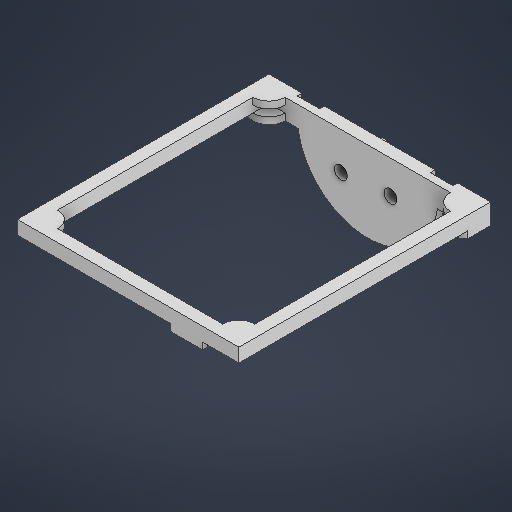
# Autodesk Inventor part: Frame
Saved by Autodesk Inventor 2026.1 (Build 301233020, 233B)
## iProperties
Created: 2026-09-21
Part Number: Frame
Material: Generic
Document SubType Name: Modeling
Designer: InventorKid
Density: 1 g/cm^3
Appearance: Default
Author: InventorKid
Autodesk Inventor part; units mm, degrees
ref_plane "YZ Plane" through (0, 0, 0) normal (1, 0, 0) x (0, 1, 0)
ref_plane "XZ Plane" through (0, 0, 0) normal (0, 1, 0) x (-1, 0, 0)
ref_plane "XY Plane" through (0, 0, 0) normal (0, 0, 1) x (1, 0, 0)
sketch "Sketch1" plane through (0, 0, 0) normal (0, 1, 0) x (-1, 0, 0)
  line L0 (0, 0) -> (48.5, 0)
  line L1 (48.5, 0) -> (48.5, 56)
  line L2 (48.5, 56) -> (0, 56)
  line L3 (0, 56) -> (0, 0)
  line L4 (48.8, 56.3) -> (48.8, -0.3)
  line L5 (48.8, -0.3) -> (-0.3, -0.3)
  line L6 (-0.3, -0.3) -> (-0.3, 56.3)
  line L7 (-0.3, 56.3) -> (48.8, 56.3)
  line L8 (51.8, 59.3) -> (51.8, -3.3)
  line L9 (51.8, -3.3) -> (-3.3, -3.3)
  line L10 (-3.3, -3.3) -> (-3.3, 59.3)
  line L11 (-3.3, 59.3) -> (51.8, 59.3)
  dimension "d0" = 56
  dimension "d1" = 48.5
  dimension "d2" = 0.3
  dimension "d3" = 3
  constraints: 24 end point, 6 parallel, 3 perpendicular, 1 horizontal, 6 other
  measures "d0" distance of L0.end L1.end
  measures "d1" distance of L1.end L2.end
  measures "d2" distance between parallel lines of L1 L4
  measures "d3" distance between parallel lines of L7 L11
extrude "Extrusion1" add sketch "Sketch1" along normal blind 1.7 contours L8 L9 L10 L11
sketch "Sketch2" plane through (0, 1.7, 0) normal (0, 1, 0) x (1, 0, 0)
  line L0 (-48.8, 0.3) -> (0.3, 0.3) projected
  line L1 (-51.8, 3.3) -> (-51.8, -59.3) projected
  line L2 (-51.8, -2.3458) -> (-51.8, 3.3)
  line L3 (-51.8, 3.3) -> (-46.1542, 3.3)
  line L4 (-2.3458, 3.3) -> (3.3, 3.3)
  arc A0 (-48.8, -3.7) -> (-44.8, 0.3) centre (-48.8, 0.3) ccw
  line L5 (3.3, -59.3) -> (3.3, 3.3) projected
  line L6 (3.3, -2.3458) -> (3.3, 3.3)
  arc A1 (-3.7, 0.3) -> (0.3, -3.7) centre (0.3, 0.3) ccw
  line L7 (0.3, -56.3) -> (-48.8, -56.3) projected
  arc A2 (-44.8, -56.3) -> (-48.8, -52.3) centre (-48.8, -56.3) ccw
  arc A3 (0.3, -52.3) -> (-3.7, -56.3) centre (0.3, -56.3) ccw
  line L8 (-51.8, -59.3) -> (3.3, -59.3) projected
  line L9 (-2.3458, -59.3) -> (3.3, -59.3)
  line L10 (3.3, -59.3) -> (3.3, -53.6542)
  line L11 (-46.1542, -59.3) -> (-51.8, -59.3)
  line L12 (-51.8, -59.3) -> (-51.8, -53.6542)
  line L13 (-48.8, -56.3) -> (-48.8, 0.3) projected
  line L14 (-44.8, 0.3) -> (-3.7, 0.3)
  line L15 (3.3, 0.3) -> (3.3, 3.3)
  line L16 (3.3, 3.3) -> (-48.8, 3.3)
  line L17 (3.3, -59.3) -> (-51.8, -59.3)
  line L18 (-51.8, -59.3) -> (-51.8, 3.3)
  line L19 (-51.8, 3.3) -> (3.3, 3.3)
  line L20 (3.3, 3.3) -> (3.3, -59.3)
  line L21 (0.3, 0.3) -> (0.3, -56.3) projected
  line L22 (-44.8, 0.3) -> (-3.7, 0.3)
  line L23 (0.3, -3.7) -> (0.3, -52.3)
  line L24 (-3.7, -56.3) -> (-44.8, -56.3)
  line L25 (-48.8, -52.3) -> (-48.8, -3.7)
  point P0 (0, 0)
  point P1 (-48.8, -3.7)
  point P2 (-48.8, -3.7)
  dimension "d8" = 4
  dimension "d9" = 4
  dimension "d14" = 8
  dimension "d15" = 8
  constraints: 38 end point, 8 point on circle, 5 horizontal, 5 parallel, 5 point on line, 4 centre point, 4 perpendicular, 2 coincident, 2 collinear, 1 vertical
  measures "d8" radius of A0
  measures "d9" radius of A1
  measures "d14" diameter of A2
  measures "d15" diameter of A3
extrude "Extrusion2" add sketch "Sketch2" along normal blind 1.7 contours L0 A0 L13 | L0 L21 A1 | A2 L7 L13 | L21 L7 A3 | L3 L16 L4 L5 L8 L1
sketch "Sketch3" plane through (0, 0, 0) normal (0, -1, 0) x (1, 0, 0)
  line L0 (-51.8, 59.3) -> (-51.8, 59.3) projected
  arc A0 (-13.7, 59.3) -> (-5.7, 59.3) centre (-9.7, 59.3) ccw
  line L1 (-13.7, 59.3) -> (-5.7, 59.3)
  arc A1 (-48.8, 52.3) -> (-44.8, 56.3) centre (-48.8, 56.3) ccw projected
  line L2 (0.3, -0.3) -> (0.3, 56.3) projected
  line L3 (3.3, -3.3) -> (-51.8, -3.3) projected
  line L4 (3.3, 59.3) -> (3.3, -3.3) projected
  line L5 (-51.8, -3.3) -> (-51.8, 59.3) projected
  arc A2 (-44.8, -0.3) -> (-48.8, 3.7) centre (-48.8, -0.3) ccw projected
  arc A3 (0.3, 3.7) -> (-3.7, -0.3) centre (0.3, -0.3) ccw projected
  line L6 (-48.8, -0.3) -> (0.3, -0.3) projected
  arc A4 (-46.1542, -3.3) -> (-51.8, 2.3458) centre (-48.8, -0.3) ccw
  arc A5 (3.3, 2.3458) -> (-2.3458, -3.3) centre (0.3, -0.3) ccw
  line L7 (-44.8, -0.3) -> (-3.7, -0.3)
  line L8 (3.3, 2.3458) -> (3.3, -3.3)
  line L9 (-51.8, -3.3) -> (-51.8, 2.3458)
  line L10 (-51.8, 59.3) -> (3.3, 59.3) projected
  dimension "d16" = 4
  dimension "d21" = 10
  constraints: 8 end point, 6 point on circle, 4 collinear, 4 point on line, 3 centre point, 2 coincident, 2 concentric, 2 midpoint, 1 horizontal, 1 other
  measures "d16" radius of A0
  measures "d21" horizontal distance of A0.centre L2.end
extrude "Extrusion3" add sketch "Sketch3" along normal blind 1.7 contours L1 A0 | A4 A2 L3 L5 | L4 L3 A5 L6 L2 | L2 L6 A3 | A4 L6 A5 L3
sketch "Sketch7" plane through (3.3, 3.4, -3.3) normal (0, 0, -1) x (-1, 0, 0)
  line L0 (55.1, -5.1) -> (0, -5.1) construction
  line L1 (0, 0) -> (55.1, 0) construction
  line L2 (55.1, -5.1) -> (0, 0) construction
  line L3 (0, -5.1) -> (55.1, 0) construction
  line L4 (45.05, -5.1) -> (10.05, -5.1)
  line L5 (10.05, -5.1) -> (10.05, 0)
  line L6 (10.05, 0) -> (45.05, 0)
  line L7 (45.05, 0) -> (45.05, -5.1)
  point P0 (3.3, -3.4)
  point P1 (27.55, -5.1)
  point P2 (27.55, -2.55)
  dimension "d39" = 35
  constraints: 12 end point, 2 collinear, 2 midpoint, 2 parallel, 1 horizontal, 1 perpendicular, 1 vertical alignment
  measures "d39" distance between parallel lines of L5 L7
extrude "Extrusion7" cut sketch "Sketch7" against normal blind 1
sketch "Sketch8" plane through (3.3, 3.4, -2.3) normal (0, 0, -1) x (-1, 0, 0)
  line L0 (45.05, 0) -> (45.05, -5.1) projected
  line L1 (10.05, -5.1) -> (10.05, 0) projected
  line L2 (45.05, -5.1) -> (10.05, 0)
  line L3 (45.05, 0) -> (55.1, 0) projected
  line L4 (45.05, -5.1) -> (10.05, -5.1) projected
  line L5 (45.05, 0) -> (10.05, -5.1)
  circle A0 centre (27.55, -2.55) radius 2
  point P0 (3.3, -3.4)
  dimension "d42" = 4
  constraints: 4 end point, 1 centre point, 1 midpoint
  measures "d42" diameter of A0
extrude "Extrusion8" add sketch "Sketch8" along normal blind 2 contours A0 L2 L5 | L5 L2 A0 | A0 L5 L2 | L5 A0 L2
sketch "Sketch9" plane through (3.3, 3.4, -2.3) normal (0, 0, -1) x (-1, 0, 0)
  circle A0 centre (34.2675, -9.2675) radius 1.6
  circle A1 centre (21.8931, -8.2069) radius 1.6
  circle A2 centre (20.8325, 4.1675) radius 1.6
  circle A3 centre (33.2069, 3.1069) radius 1.6
  line L0 (34.2675, -9.2675) -> (20.8325, 4.1675)
  line L1 (33.2069, 3.1069) -> (21.8931, -8.2069)
  circle A4 centre (27.55, -2.55) radius 17.5
  circle A5 centre (27.55, -2.55) radius 2 projected
  line L2 (27.55, -2.55) -> (10.05, -2.55)
  line L3 (45.05, 0) -> (55.1, 0) projected
  line L4 (45.05, 0) -> (10.05, 0)
  line L5 (7, -5.1) -> (48.1, -5.1) projected
  line L6 (45.05, -5.1) -> (10.05, -5.1)
  line L7 (10.05, -5.1) -> (10.05, 0)
  line L8 (10.05, 0) -> (45.05, 0)
  line L9 (45.05, 0) -> (45.05, -5.1)
  point P0 (3.3, -3.4)
  point P1 (25.55, -2.55)
  point P2 (44.8632, 0)
  point P3 (30.1, 0)
  point P4 (28.9642, -1.1358)
  point P5 (10.2368, 0)
  point P6 (10.05, -5.1)
  point P7 (10.2368, -5.1)
  point P8 (45.05, -2.55)
  point P9 (44.8632, -5.1)
  dimension "d47" = 35
  dimension "d45" = 19
  dimension "d46" = 16
  dimension "d48" = 45
  dimension "d49" = 3.2
  constraints: 16 end point, 4 centre point, 3 equal radius, 3 horizontal, 2 midpoint, 2 parallel, 2 perpendicular, 1 coincident, 1 point on line, 4 other
  measures "d45" distance of L0.start L0.end
  measures "d46" distance of L1.start L1.end
  measures "d48" angle of L2 L1
  measures "d49" diameter of A0
extrude "Extrusion9" add sketch "Sketch9" along normal blind 1 and the other way blind 2 contours L5 L1 A5 L0 | L5 A4 | L0 A5 L1 L4 A4 L5 | A5 L1 L0 | L0 L1 A5 | L5 A4 L2 A5 L1 | A4 L9 L5 | L2 A5 L0 | L0 A5 L1 | L1 A5 L2 | L5 L7 A4 | A4 L4 L9 | A5 L2 A4 L4 L0 | L0 L4 L1 A5 | L7 L4 A4
sketch "Sketch10" plane through (3.3, 3.4, -3.3) normal (0, 0, -1) x (-1, 0, 0)
  circle A0 centre (27.55, -2.55) radius 14
  circle A1 centre (27.55, -2.55) radius 19.5
  circle A2 centre (27.55, -2.55) radius 2 projected
  point P0 (3.3, -3.4)
  dimension "d54" = 39
  dimension "d55" = 28
  constraints: 2 centre point, 1 coincident, 1 concentric
  measures "d54" diameter of A1
  measures "d55" diameter of A0
extrude "Extrusion10" cut sketch "Sketch10" against normal blind 1.2 contours A1
equation "\"d7\" = d6"
equation "\"d6\" = 8"
body "Solid1"
